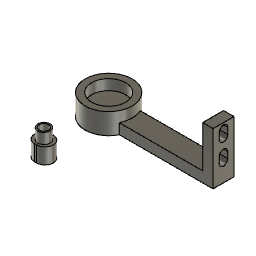
Roulement volet SAE (Autodesk Fusion 360 design; units mm, degrees)
Autodesk Fusion 360 part; units mm, degrees
sketch "Esquisse1" plane through (0, 0, 0) normal (0, 0, 1) x (1, 0, 0)
  line L0 (8, -8) -> (10, -8)
  arc A0 (10, -8) -> (10, 8) centre (10, 0) ccw
  line L1 (10, 8) -> (8, 8)
  arc A1 (8, 8) -> (8, -8) centre (8, 0) ccw
  line L2 (0, 0) -> (18, 0) construction
  circle A2 centre (9, 0) radius 2.75
  dimension "d1" = 16
  dimension "d2" = 5.5
  dimension "d29" = 18
  constraint tangent L0 A0
  constraint tangent A0 L1
  constraint parallel L0 L1
  constraint tangent L1 A1
  constraint tangent L0 A1
  constraint midpoint A1 L2.start
  constraint midpoint A0 L2.end
  constraint horizontal L2
  constraint coincident L2.start origin
  constraint midpoint L2 A2.centre
  measures "d1" diameter of A0
  measures "d2" diameter of A2
  measures "d29" distance of L2.start L2.end
extrude "Extrusion1" add sketch "Esquisse1" along normal blind 15 makes body 1
thread "Filetage1" "ISO Metric profile 5.5 M5.5x0.5 6H" major diameter 5.5961 minor diameter 5.0287 pitch 0.5 angle 60 resizes the face on face at (11.7363, -0.2738, 10) on bodies 1
sketch "Esquisse2" plane through (0, 0, 15) normal (0, 0, 1) x (-1, 0, 0)
  circle A0 centre (-9, 0) radius 2.5143
  arc A1 (-8, -8) -> (-8, 8) centre (-8, 0) ccw
  line L0 (-8, 8) -> (-10, 8)
  arc A2 (-10, 8) -> (-10, -8) centre (-10, 0) ccw
  line L1 (-10, -8) -> (-8, -8)
  circle A3 centre (-9, 0) radius 5.925
  dimension "d13" = 11.85
  constraint concentric A0 A3
  measures "d13" diameter of A3
extrude "Extrusion2" add sketch "Esquisse2" along normal blind 10 contours A3 bodies 1
hole "Perçage1" at (9, 0, 25) direction (0, 0, -1) diameter 5.5 depth 7 tip angle 180 counterbore diameter 9 counterbore depth 7 bodies 1
sketch "Esquisse3" plane through (0, 0, 0) normal (0, 0, 1) x (1, 0, 0)
  circle A0 centre (6, 40) radius 16.25
  circle A1 centre (6, 40) radius 22.5
  dimension "d12" = 32.5
  dimension "d14" = 45
  constraint concentric A0 A1
extrude "Extrusion3" add sketch "Esquisse3" along normal blind 10 separate body makes body 2
sketch "Esquisse4" plane through (0, 0, 10) normal (0, 0, 1) x (-1, 0, 0)
  circle A0 centre (-6, -40) radius 16.25
  circle A1 centre (-6, -40) radius 22.5
  line L0 (-6, -50) -> (-116, -50)
  line L1 (-116, -50) -> (-116, -30)
  line L2 (-116, -30) -> (-6, -30)
  line L3 (-6, -30) -> (-6, -50)
  dimension "d17" = 110
  dimension "d20" = 10
  dimension "d21" = 20
  constraint horizontal L0
  constraint vertical L1
  constraint horizontal L2
  constraint vertical L3
  measures "d17" distance of L0.start L0.end
  measures "d21" distance of L0.start L2.end
extrude "Extrusion4" add sketch "Esquisse4" along normal blind 10 bodies 2
sketch "Esquisse5" plane through (0, 0, 20) normal (0, 0, 1) x (-1, 0, 0)
  arc A0 (-26.1556, -50) -> (-26.1556, -30) centre (-6, -40) ccw
  line L0 (-26.1556, -30) -> (-116, -30)
  line L1 (-116, -30) -> (-116, -50)
  line L2 (-116, -50) -> (-26.1556, -50)
  line L3 (-116, -50) -> (-106, -50)
  line L4 (-106, -50) -> (-106, -30)
  line L5 (-106, -30) -> (-116, -30)
  line L6 (-116, -30) -> (-116, -50)
  dimension "d22" = 10
  constraint horizontal L3
  constraint vertical L4
  constraint horizontal L5
  constraint vertical L6
  constraint coincident L1.end L2.start
  measures "d22" distance of L1.end L3.end
extrude "Extrusion5" add sketch "Esquisse5" along normal blind 40 contours L0 L1 L2 L3 L4 L5 L6 bodies 2
sketch "Esquisse6" plane through (106, 0, 0) normal (-1, 0, 0) x (0, -1, 0)
  line L0 (-50, 20) -> (-30, 20)
  line L1 (-30, 20) -> (-30, 60)
  line L2 (-30, 60) -> (-50, 60)
  line L3 (-50, 60) -> (-50, 20)
  line L4 (-44.125, 54) -> (-44.125, 48)
  arc A0 (-44.125, 48) -> (-35.875, 48) centre (-40, 48) ccw
  line L5 (-35.875, 48) -> (-35.875, 54)
  arc A1 (-35.875, 54) -> (-44.125, 54) centre (-40, 54) ccw
  line L6 (-40, 54) -> (-40, 48) construction
  line L7 (-44.125, 34) -> (-44.125, 28)
  arc A2 (-44.125, 28) -> (-35.875, 28) centre (-40, 28) ccw
  line L8 (-35.875, 28) -> (-35.875, 34)
  arc A3 (-35.875, 34) -> (-44.125, 34) centre (-40, 34) ccw
  line L9 (-40, 34) -> (-40, 28) construction
  line L10 (-40, 60) -> (-40, 20) construction
  dimension "d25" = 8.25
  dimension "d26" = 8.25
  dimension "d35" = 6
  dimension "d36" = 6
  constraint tangent L4 A0
  constraint tangent A0 L5
  constraint parallel L4 L5
  constraint tangent L5 A1
  constraint tangent L4 A1
  constraint vertical L6
  constraint tangent L7 A2
  constraint tangent A2 L8
  constraint parallel L7 L8
  constraint tangent L8 A3
  constraint tangent L7 A3
  constraint parallel L3 L9
  constraint midpoint L2 L10.start
  constraint midpoint L0 L10.end
  measures "d25" diameter of A0
  measures "d26" diameter of A2
  measures "d35" distance of A3.centre A2.centre
  measures "d36" distance of A1.centre A0.centre
extrude "Extrusion6" cut sketch "Esquisse6" against normal blind 10 contours L4 A0 L5 A1 | L7 A2 L8 A3 bodies 2
sketch "Esquisse7" plane through (0, 0, 0) normal (0, 0, -1) x (1, 0, 0)
  circle A0 centre (9, 0) radius 2.5143
  arc A1 (8, 8) -> (8, -8) centre (8, 0) ccw
  line L0 (8, -8) -> (10, -8)
  arc A2 (10, -8) -> (10, 8) centre (10, 0) ccw
  line L1 (10, 8) -> (8, 8)
  ellipse E0 centre (9, 0) end of major axis (16.5, 0) minor radius 6.5
  line L2 (1.5, 0) -> (16.5, 0) construction
  line L3 (9, -6.5) -> (9, 6.5) construction
  dimension "d30" = 13
  dimension "d33" = 15
  constraint coincident E0 L2.start
  constraint coincident E0 L2.end
  constraint coincident E0 L3.start
  constraint coincident E0 L3.end
  constraint concentric A0 E0
  constraint horizontal L2
  measures "d33" distance of E0
extrude "Extrusion7" cut sketch "Esquisse7" against normal blind 4 contours E0 bodies 1
ref_plane "Plan de construction1" through (81, 40, 40) normal (-1, 0, 0) x (0, -1, 0)
split "Scinder1" by plane through (81, 40, 40) normal (-1, 0, 0) bodies 2 makes body 3 at (44.4371, 43.3333, 20)
move_body "Déplacer1" bodies 2 to x (1, 0, 0) y (0, -1, 0) z (0, 0, -1) at (0, 80, 30)
fillet "Congé1" radius 2 8 edges at (106, 40, 6.125) (106, 35.875, -1) (106, 40, -8.125) (106, 44.125, -1) (106, 40, -13.875) (106, 35.875, -21) (106, 40, -28.125) (106, 44.125, -21) on bodies 2
combine "Combiner1" operation add target body 3 tool bodies 2
move_body "Déplacer2" bodies 3 to x (1, 0, 0) y (0, -1, 0) z (0, 0, -1) at (0, 105, 20)
named bodies: "Bout volet", "Patte_attache", "Patte_roulement"
